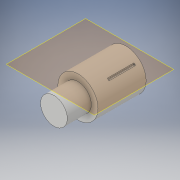
# Autodesk Inventor part: 軸1
Saved by Autodesk Inventor 2019 (Build 230136000, 136)
## iProperties
Created: 2019-12-29
Part Number: 軸1
Material: 一般
Document SubType Name: Modeling
Designer: Dorian Liu
Density: 1 g/cm^3
Appearance: 預設
Author: Dorian Liu
Autodesk Inventor part; units mm, degrees
ref_plane "YZ Plane" through (0, 0, 0) normal (1, 0, 0) x (0, 1, 0)
ref_plane "XY Plane" through (0, 0, 0) normal (0, 0, 1) x (1, 0, 0)
sketch "草圖2" plane through (0, 0, 0) normal (0, 0, 1) x (1, 0, 0)
  circle A0 centre (0, 0) radius 7.5
  dimension "d3" = 15
  constraints: 1 centre point, 1 coincident
  measures "d3" diameter of A0
extrude "擠出2" add sketch "草圖2" along normal blind 18
sketch "草圖3" plane through (0, 0, 18) normal (0, 0, 1) x (1, 0, 0)
  circle A0 centre (0, 0) radius 5
  dimension "d6" = 10
  constraints: 1 centre point, 1 coincident
  measures "d6" diameter of A0
extrude "擠出3" add sketch "草圖3" along normal blind 9
ref_plane "工作平面2" through (0, 7.5, 0) normal (0, 1, 0) x (-1, 0, 0)
sketch "草圖5" plane through (0, 7.5, 0) normal (0, 1, 0) x (-1, 0, 0)
  line L0 (-5, 12) -> (-10, 12)
  line L1 (-10, 12) -> (-10, 2)
  line L2 (-10, 2) -> (-5, 2)
  line L3 (-5, 2) -> (-5, 12)
  line L4 (-7.5, 0) -> (7.5, 0) projected
  point P0 (0, 0)
  dimension "d16" = 5
  dimension "d17" = 10
  dimension "d18" = 2
  dimension "d19" = 12.5
  constraints: 8 end point, 2 parallel, 1 horizontal, 1 perpendicular
  measures "d16" distance of L2.end L1.end
  measures "d17" distance of L1.end L0.end
  measures "d18" distance between parallel lines of L4 L2
  measures "d19" distance from line of L4.end L3
extrude "擠出5" cut sketch "草圖5" against normal blind 2.5
fillet "圓角1" radius 0.16 3 edges at (5, 5, 7) (5.2951, 5, 12) (5.2951, 5, 2)
fillet "圓角2" radius 0.16 4 edges at (5.0469, 5.0469, 11.9531) (5, 5.3751, 12) (5.0469, 5.0469, 2.0469) (5, 5.3751, 2)
